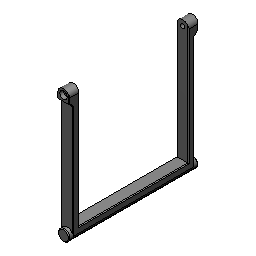
Adjustable_Angle_Bar (Autodesk Fusion 360 design; units mm, degrees)
Autodesk Fusion 360 part; units mm, degrees
note: some values were not read from the file. Chosen so that the rebuilt part matches the saved one: which pieces of a blend or face edit are solid.
sketch "Sketch1" plane through (0, 0, 0) normal (0, 1, 0) x (1, 0, 0)
  circle A0 centre (0, 0) radius 1.75
  circle A1 centre (0, 0) radius 3
  circle A2 centre (0, 0) radius 4.65
  line L0 (-4.65, 0) -> (-4.65, 100)
  line L1 (4.65, 0) -> (4.65, 100)
  circle A3 centre (0, 100) radius 4.65
  line L2 (4.65, 4.65) -> (-4.65, 4.65)
  dimension "d1" = 3.5
  dimension "d2" = 6
  dimension "d3" = 9.3
  dimension "d4" = 100
  constraint coincident A0.centre A1.centre
  constraint concentric A1 A2
  constraint coincident A2 L0.start
  constraint vertical L0
  constraint horizontal A0.centre L0.start
  constraint coincident A2 L1.start
  constraint tangent A2 L1
  constraint parallel L0 L1
  constraint coincident L0.end A3
  constraint tangent L0 A3
  constraint coincident L1.end A3
  constraint tangent L1 A3
  constraint coincident L1 L2.start
  constraint coincident L0 L2.end
  constraint perpendicular L0 L2
  constraint tangent A2 L2
  measures "d1" diameter of A0
  measures "d2" diameter of A1
  measures "d3" diameter of A2
  measures "d4" distance of L0.start L0.end
extrude "Extrude1" add sketch "Sketch1" along normal blind 8 contours A2 | A2 L0 L2 | A2 L1 L2 | A3 makes body 1 at (2.9963, 5.3333, 0.1495) makes body 2 at (4.6442, 2.6667, -99.7682)
extrude "Extrude2" add sketch "Sketch1" along normal blind 5 contours A1 | A2 L0 L2 | A2 L1 L2 | L0 L1 A3 L2 bodies 1 2
chamfer "Chamfer1" distance 3 angle 45 1 edges at (0, 5, -4.65) on bodies 1
sketch "Sketch2" plane through (0, 0, 0) normal (0, -1, 0) x (1, 0, 0)
  circle A0 centre (0, 0) radius 1.75
  arc A1 (4.65, 0) -> (-4.65, 0) centre (0, 0) ccw
  line L0 (-4.65, 0) -> (-4.65, -100)
  arc A2 (-4.65, -100) -> (4.65, -100) centre (0, -100) ccw
  line L1 (4.65, -100) -> (4.65, 0)
  circle A3 centre (0, -100) radius 4.65
  line L2 (-4.65, -95.35) -> (4.65, -95.35)
  constraint coincident L0 L2.start
  constraint coincident L1 L2.end
  constraint perpendicular L1 L2
  constraint tangent A3 L2
extrude "Extrude3" add sketch "Sketch2" along normal blind 45 contours L1 A3 L2 | L0 A3 L2 | A2 A3 bodies 1
mirror "Mirror1" about plane through (0, -45, 0) normal (0, -1, 0) of bodies 1 merged
chamfer "Chamfer2" distance 0.6 angle 45 1 faces at (4.65, 1.6667, -34.3331) on bodies 1
chamfer "Chamfer3" distance 0.6 angle 45 2 edges at (-4.3353, 8, -98.3185) (-4.3353, -98, -98.3185) on bodies 1
equation "d3 = ( 4.65 * 2 ) * 1 mm"
equation "d4 = BarLength"
equation "BarLength = 100 mm"
